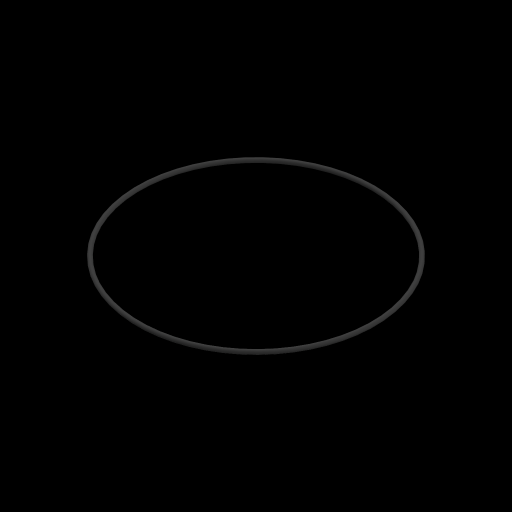
# Autodesk Inventor part: OringV1
Saved by Autodesk Inventor 2024 (Build 280153000, 153)
## iProperties
Created: 2026-04-12
Part Number: OringV1
Material: Generic
Document SubType Name: Modeling
Designer: Tanner
Density: 1 g/cm^3
Appearance: Rubber - Black
Author: Tanner
Autodesk Inventor part; units mm, degrees
ref_plane "YZ Plane" through (0, 0, 0) normal (1, 0, 0) x (0, 1, 0)
ref_plane "XZ Plane" through (0, 0, 0) normal (0, 1, 0) x (-1, 0, 0)
ref_plane "XY Plane" through (0, 0, 0) normal (0, 0, 1) x (1, 0, 0)
sketch "Sketch1" plane through (0, 0, 0) normal (0, 0, 1) x (1, 0, 0)
  line L0 (-100, 0) -> (-96.5, 0) construction
  line L1 (-96.5, 0) -> (-96.5, 3.5) construction
  line L2 (-96.5, 3.5) -> (-100, 3.5) construction
  line L3 (-100, 3.5) -> (-100, 0) construction
  line L4 (-100, 0) -> (-96.5, 3.5) construction
  line L5 (-96.5, 0) -> (-100, 3.5) construction
  circle A0 centre (-98.25, 1.75) radius 1.75
  line L6 (0, -0.7) -> (0, 4.2) projected
  point P0 (0, 0)
  dimension "d3" = 3.5
  dimension "d4" = 3.5
  dimension "d5" = 96.5
  constraints: 12 end point, 2 midpoint, 2 parallel, 1 centre point, 1 coincident, 1 horizontal, 1 horizontal alignment, 1 perpendicular, 1 tangent
  measures "d3" distance of L2.end L1.end
  measures "d4" distance of L1.end L0.end
  measures "d5" distance from line of point (0, 0) L1
revolve "Revolution1" add sketch "Sketch1" angle 360 about axis through (0, -10, 0) along (0, 1, 0)
body "Solid1"
